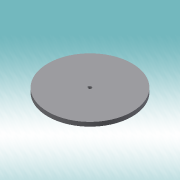
# Autodesk Inventor part: 計測輪
Saved by Autodesk Inventor 2015 (Build 190159000, 159)
## iProperties
Created: 2016-03-11
Part Number: 計測輪
Material: 一般
Document SubType Name: Modeling
Designer: buzztaka
Density: 1 g/cm^3
Appearance: 既定
Author: buzztaka
Autodesk Inventor part; units mm, degrees
ref_plane "YZ Plane" through (0, 0, 0) normal (1, 0, 0) x (0, 1, 0)
ref_plane "XZ Plane" through (0, 0, 0) normal (0, 1, 0) x (-1, 0, 0)
ref_plane "XY Plane" through (0, 0, 0) normal (0, 0, 1) x (1, 0, 0)
sketch "スケッチ1" plane through (0, 0, 0) normal (0, 0, 1) x (1, 0, 0)
  circle A0 centre (0, 0) radius 152
  dimension "d0" = 304
  constraints: 1 centre point, 1 coincident
  measures "d0" diameter of A0
extrude "押し出し1" add sketch "スケッチ1" along normal blind 15
sketch "スケッチ2" plane through (0, 0, 0) normal (0, 0, -1) x (-1, 0, 0)
  point P0 (0, 0)
  point P1 (0, 0)
  constraints: 1 coincident
hole "穴1" at (0, 0, 0) direction (0, 0, 1) diameter 12 end through all
sketch "スケッチ3" plane through (0, 0, 0) normal (0, 0, -1) x (-1, 0, 0)
  circle A0 centre (0, 0) radius 6 projected
sketch "スケッチ4" plane through (0, 0, 15) normal (0, 0, 1) x (1, 0, 0)
  line L0 (-7.8, -2) -> (-2.8778, -2)
  line L1 (-2.8778, -2) -> (-2.8778, 2)
  line L2 (-2.8778, 2) -> (-7.8, 2)
  line L3 (-7.8, 2) -> (-7.8, -2)
  point P0 (0, 0)
  point P1 (-7.8, 0)
  dimension "d10" = 7.8
  dimension "d11" = 2
  dimension "d12" = 2
  constraints: 8 end point, 2 parallel, 1 horizontal, 1 perpendicular
  measures "d10" distance of point (0, 0) point (-7.8, 0)
  measures "d11" distance of point (-7.8, 0) point (-7.8, 2)
  measures "d12" distance of L0.start point (-7.8, 0)
extrude "押し出し2" cut sketch "スケッチ4" against normal blind 20
